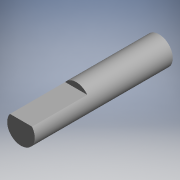
# Autodesk Inventor part: shaft
Saved by Autodesk Inventor 2019.4 (Build 234330000, 330)
## iProperties
Created: 2020-06-20
Part Number: shaft
Material: Generic
Document SubType Name: Modeling
Designer: Jorge
Density: 1 g/cm^3
Appearance: Default
Author: Jorge
Autodesk Inventor part; units mm, degrees
ref_plane "YZ Plane" through (0, 0, 0) normal (1, 0, 0) x (0, 1, 0)
ref_plane "XZ Plane" through (0, 0, 0) normal (0, 1, 0) x (-1, 0, 0)
ref_plane "XY Plane" through (0, 0, 0) normal (0, 0, 1) x (1, 0, 0)
sketch "Sketch1" plane through (0, 0, 0) normal (0, 0, 1) x (1, 0, 0)
  arc A0 (-2, 1.5) -> (2, 1.5) centre (0, 0) ccw
  line L0 (-2, 1.5) -> (2, 1.5)
  arc A1 (2, 1.5) -> (-2, 1.5) centre (0, 0) ccw
  dimension "d0" = 5
  dimension "d1" = 4
  constraints: 4 point on circle, 2 centre point, 2 end point, 1 coincident, 1 horizontal
  measures "d0" diameter of A0
extrude "Extrusion1" add sketch "Sketch1" along normal blind 10 contours L0 A0
extrude "Extrusion2" add sketch "Sketch1" against normal blind 15
body "Solid1"
